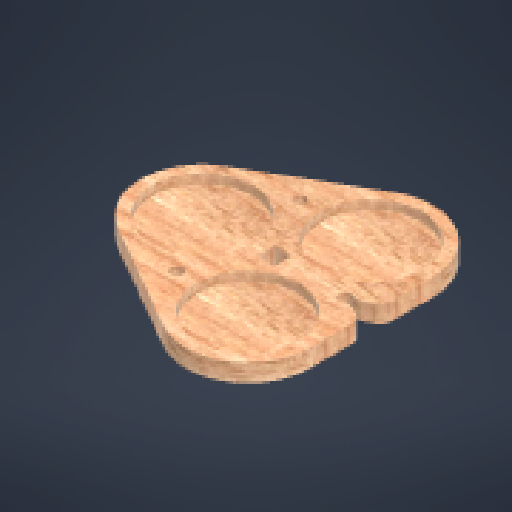
# Autodesk Inventor part: TOP_PLATE_WEIGHTS_TREBUCHET
Saved by Autodesk Inventor 2026.2 (Build 302298010, 298A)
## iProperties
Created: 2026-02-19
Part Number: TOP_PLATE_WEIGHTS_TREBUCHET
Material: Wood (Birch)
Document SubType Name: Modeling
Designer: 4aida
Density: 0.55 g/cm^3
Appearance: Birch - Natural Polished
Mass: 41.5218 g
Surface Area: 304.408 cm^2
Volume: 75.4942 cm^3
Author: 4aida
Autodesk Inventor part; units mm, degrees
ref_plane "YZ Plane" through (0, 0, 0) normal (1, 0, 0) x (0, 1, 0)
ref_plane "XZ Plane" through (0, 0, 0) normal (0, 1, 0) x (-1, 0, 0)
ref_plane "XY Plane" through (0, 0, 0) normal (0, 0, 1) x (1, 0, 0)
sketch "Sketch1" plane through (0, 0, 0) normal (0, 1, 0) x (-1, 0, 0)
  line L0 (54.5331, -28.5412) -> (-2.5492, -61.4977)
  line L1 (-51.9839, -32.9565) -> (-51.9839, 32.9565)
  line L2 (-2.5492, 61.4977) -> (54.5331, 28.5412)
  circle A0 centre (38.0549, 0) radius 32.9565 construction
  circle A1 centre (-19.0274, 32.9565) radius 32.9565 construction
  circle A2 centre (-19.0274, -32.9565) radius 32.9565 construction
  line L3 (4.7625, -4.7625) -> (-4.7625, -4.7625)
  line L4 (-4.7625, -4.7625) -> (-4.7625, 4.7625)
  line L5 (-4.7625, 4.7625) -> (4.7625, 4.7625)
  line L6 (4.7625, 4.7625) -> (4.7625, -4.7625)
  line L7 (4.7625, -4.7625) -> (-4.7625, 4.7625) construction
  line L8 (-4.7625, -4.7625) -> (4.7625, 4.7625) construction
  line L9 (-51.9839, 4.875) -> (-48.5839, 4.875)
  line L10 (-48.5839, 4.875) -> (-40.8685, 1.3266)
  line L11 (-40.8685, -1.3266) -> (-48.5839, -4.875)
  line L12 (-48.5839, -4.875) -> (-51.9839, -4.875)
  arc A3 (54.5331, -28.5412) -> (54.5331, 28.5412) centre (38.0549, 0) ccw
  arc A4 (-2.5492, 61.4977) -> (-51.9839, 32.9565) centre (-19.0274, 32.9565) ccw
  arc A5 (-51.9839, -32.9565) -> (-2.5492, -61.4977) centre (-19.0274, -32.9565) ccw
  arc A6 (-40.8685, -1.3266) -> (-40.8685, 1.3266) centre (-37.9839, 0) ccw
  line L13 (-37.9839, 0) -> (-40.8685, -1.3266) construction
  line L14 (-37.9839, 0) -> (-40.8685, 1.3266) construction
  arc A7 (21.5831, -34.7299) -> (19.2854, -36.0565) centre (18.992, -32.8951) ccw
  arc A8 (19.2854, 36.0565) -> (21.5831, 34.7299) centre (18.992, 32.8951) ccw
  circle A9 centre (18.992, 32.8951) radius 3.175
  circle A10 centre (18.992, -32.8951) radius 3.175
  point P0 (0, 0)
  point P1 (0, 0)
  point P2 (-51.9839, 0)
  point P3 (21.5831, 34.7299)
  point P4 (21.5831, -34.7299)
  dimension "d0" = 9.525
  dimension "d1" = 9.525
  dimension "d2" = 65.913
  dimension "d5" = 14
  dimension "d6" = 3.4
  dimension "d7" = 9.75
  dimension "d12" = 6.35
  dimension "d15" = 360
  constraints: 30 end point, 18 point on circle, 9 centre point, 9 tangent, 4 coincident, 3 concentric, 3 midpoint, 2 collinear, 2 horizontal, 2 horizontal alignment, 2 parallel, 2 perpendicular, 2 point on line, 1 equal length, 1 vertical alignment, 23 other
  measures "d0" distance of L4.end L5.end
  measures "d1" distance of L3.end L4.end
  measures "d2" diameter of A1
  measures "d5" distance from line of L1 point (-37.984, 0)
  measures "d6" distance of L9.start L9.end
  measures "d7" distance between parallel lines of L12 L9
  measures "d12" diameter of A6
extrude "Extrusion1" add sketch "Sketch1" along normal blind 9.525 contours L0 A5 L1 L12 L11 A6 L10 L9 A4 L2 A3
fillet "Fillet1" radius 6.35 7 edges at (51.9839, 4.7625, 4.875) (51.9839, 4.7625, -4.875) (51.9839, 4.7625, 32.9565) (-54.5331, 4.7625, -28.5412) (51.9839, 4.7625, -32.9565) (40.8685, 4.7625, 1.3266) (40.8685, 4.7625, -1.3266)
sketch "Sketch2" plane through (0, 9.525, 0) normal (0, 1, 0) x (1, 0, 0)
  circle A0 centre (19.0274, -32.9565) radius 32.9565
  circle A1 centre (19.0274, -32.9565) radius 26.9875
  circle A2 centre (19.0274, 32.9565) radius 32.9565
  circle A3 centre (19.0274, 32.9565) radius 26.9875
  circle A4 centre (-38.0549, 0) radius 32.9565
  circle A5 centre (-38.0549, 0) radius 26.9875
  line L0 (-54.5331, -28.5412) -> (2.5492, -61.4977) projected
  line L1 (2.5492, 61.4977) -> (-54.5331, 28.5412) projected
  line L2 (51.9839, -32.9565) -> (51.9839, 32.9565) projected
  line L3 (51.9839, -32.9565) -> (51.9839, 32.9565) projected
  point P0 (0, 0)
  point P1 (-94.4429, -5.4993)
  point P2 (42.4589, -84.5396)
  point P3 (42.4589, 84.5396)
  point P4 (-94.4429, 5.4993)
  point P5 (51.9839, 10.4982)
  point P6 (51.9839, 79.0403)
  point P7 (51.9839, -79.0403)
  point P8 (51.9839, -10.4982)
  point P9 (2.5492, 61.4977)
  point P10 (-54.5331, 28.5412)
  point P11 (-9.5137, 16.4782)
  point P12 (-54.5331, -28.5412)
  point P13 (2.5492, -61.4977)
  point P14 (-9.5137, -16.4783)
  point P15 (19.0274, 0)
  dimension "d9" = 53.975
  constraints: 9 tangent, 6 centre point, 3 coincident, 2 equal radius
  measures "d9" diameter of A5
extrude "Extrusion2" cut sketch "Sketch2" against normal blind 5 contours A1 | A3 | A5
body "Solid1"
